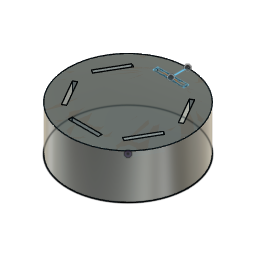
lightbox-base (Autodesk Fusion 360 design; units mm, degrees)
Autodesk Fusion 360 part; units mm, degrees
sketch "Base of Circle" plane through (0, 0, 0) normal (0, 0, 1) x (1, 0, 0) in component "Base"
  circle A0 centre (0, 0) radius 100
  dimension "d1" = 200
  constraint coincident A0.centre origin
  measures "d1" diameter of A0
extrude "Extrude1" add sketch "Base of Circle" along normal blind 75 in component "Base"
sketch "First Hole for Acrylic" plane through (0, 0, 75) normal (0, 0, 1) x (-1, 0, 0) in component "Base"
  circle A0 centre (0, 0) radius 100
  line L0 (0, -100) -> (0, -75)
  line L1 (0, -75) -> (0, -71.825)
  line L2 (25, -68.65) -> (-25, -68.65)
  line L3 (-25, -68.65) -> (-25, -75)
  line L4 (-25, -75) -> (25, -75)
  line L5 (25, -75) -> (25, -68.65)
  line L6 (25, -68.65) -> (-25, -75) construction
  line L7 (-25, -68.65) -> (25, -75) construction
  point P0 (0, -71.825)
  dimension "d4" = 25
  dimension "d6" = 3.175
  dimension "d7" = 50
  dimension "d8" = 6.35
  constraint coincident A0 L0.start
  constraint vertical L0
  constraint parallel L0 L1
  constraint horizontal L2
  constraint perpendicular L2 L3
  constraint parallel L2 L4
  constraint parallel L3 L5
  constraint coincident L6 P0
  constraint coincident L7 P0
  constraint coincident P0 L1.end
  measures "d4" distance of L0.start L0.end
  measures "d6" distance of L0.end P0
  measures "d7" distance of L3.end L4.end
  measures "d8" distance of L2.end L3.end
extrude "Extrude2" cut sketch "First Hole for Acrylic" against normal blind 25 contours L2 L3 L4 L5 in component "Base"
pattern_circular "C-Pattern1" count 6 over 360 about axis through (0, 0, 1.75) along (0, 0, 1) of "Extrude2" in component "Base"
shell "Shell1" thickness 20 removed faces 1 at (-27.1036, -4.9681, 0) in component "Base"
sketch "Acrylic Slot" plane through (0, 0, 50) normal (0, 0, 1) x (-1, 0, 0)
  line L0 (-77.4519, 15.8493) -> (-71.9527, 12.6743)
  line L1 (-71.9527, 12.6743) -> (-46.9527, 55.9756)
  line L2 (-46.9527, 55.9756) -> (-52.4519, 59.1506)
  line L3 (-52.4519, 59.1506) -> (-77.4519, 15.8493)
sketch "Wire Hole" plane through (0, 0, 50) normal (0, 0, 1) x (-1, 0, 0)
  line L0 (-49.5597, 51.467) -> (-55.1, 54.6) construction
  circle A0 centre (-52.3299, 53.0335) radius 3
  circle A1 centre (-72.0933, -18.8022) radius 3
  circle A2 centre (-19.7634, -71.8357) radius 3
  circle A3 centre (52.3299, -53.0335) radius 3
  circle A4 centre (72.0933, 18.8022) radius 3
  circle A5 centre (19.7634, 71.8357) radius 3
  dimension "d14" = 6
  dimension "d16" = 360
  constraint midpoint L0 A0.centre
  measures "d14" diameter of A0
extrude "Extrude3" cut sketch "Wire Hole" against normal blind 25 in component "Base"
component "Lightbox" placed x (1, 0, 0) y (0, 1, 0) z (0, 0, 1) at (0, 0, 0)
component "Base" placed x (1, 0, 0) y (0, 1, 0) z (0, 0, 1) at (0, 0, 0) in component "Lightbox"
equation "Acrylic_Thickness = ( 1 / 4 ) * 1 in"
equation "d6 = Acrylic_Thickness / 2"
equation "d8 = Acrylic_Thickness"
